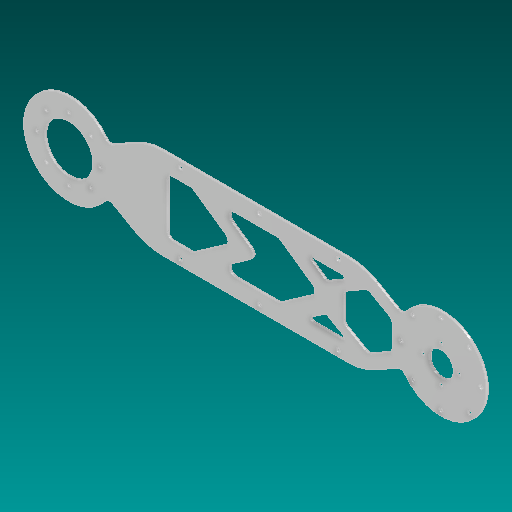
# Autodesk Inventor part: arm1 tweede kant
Saved by Autodesk Inventor 2020.3 (Build 243373000, 373)
## iProperties
Created: 2020-05-23
Part Number: arm1 tweede kant
Material: Aluminum 6061
Document SubType Name: Sheet Metal
Designer: Svend
Mass: 232.394 g
Surface Area: 513.63 cm^2
Volume: 86.0718 cm^3
Density: 2.7 g/cm^3
Sheet Metal Rule: Default_mm
Appearance: Aluminum - Polished
Author: Svend
Autodesk Inventor part; units mm, degrees
ref_plane "YZ Plane" through (0, 0, 0) normal (1, 0, 0) x (0, 1, 0)
ref_plane "XZ Plane" through (0, 0, 0) normal (0, 1, 0) x (-1, 0, 0)
ref_plane "XY Plane" through (0, 0, 0) normal (0, 0, 1) x (1, 0, 0)
sketch "Sketch1" plane through (0, 0, 0) normal (0, 0, 1) x (1, 0, 0)
  circle A0 centre (346.0004, 0) radius 1.55
  circle A1 centre (330, 0) radius 11
  arc A2 (51.9261, 10.7279) -> (51.9261, 14.7279) centre (51.9261, 12.7279) ccw
  line L0 (51.9261, 10.7279) -> (41.9261, 10.7279)
  arc A3 (41.9261, 14.7279) -> (41.9261, 10.7279) centre (41.9261, 12.7279) ccw
  line L1 (41.9261, 14.7279) -> (51.9261, 14.7279)
  arc A4 (77.3819, 10.7279) -> (77.3819, 14.7279) centre (77.3819, 12.7279) ccw
  line L2 (77.3819, 10.7279) -> (67.3819, 10.7279)
  arc A5 (67.3819, 14.7279) -> (67.3819, 10.7279) centre (67.3819, 12.7279) ccw
  line L3 (67.3819, 14.7279) -> (77.3819, 14.7279)
  arc A6 (51.9261, -14.7279) -> (51.9261, -10.7279) centre (51.9261, -12.7279) ccw
  line L4 (51.9261, -14.7279) -> (41.9261, -14.7279)
  arc A7 (41.9261, -10.7279) -> (41.9261, -14.7279) centre (41.9261, -12.7279) ccw
  line L5 (41.9261, -10.7279) -> (51.9261, -10.7279)
  arc A8 (67.3819, -10.7279) -> (67.3819, -14.7279) centre (67.3819, -12.7279) ccw
  line L6 (67.3819, -10.7279) -> (77.3819, -10.7279)
  arc A9 (77.3819, -14.7279) -> (77.3819, -10.7279) centre (77.3819, -12.7279) ccw
  line L7 (77.3819, -14.7279) -> (67.3819, -14.7279)
  circle A10 centre (59.654, 0) radius 8.5
  circle A11 centre (28, 0) radius 1.6
  line L8 (0, -40) -> (330, -40)
  arc A12 (330, -40) -> (330, 40) centre (330, 0) ccw
  line L9 (330, 40) -> (0, 40)
  arc A13 (0, 40) -> (0, -40) centre (0, 0) ccw
  line L10 (-4.8, -1) -> (-4.8, 1)
  line L11 (-4.8, 1) -> (-3.873, 1)
  arc A14 (-3.873, -1) -> (-3.873, 1) centre (0, 0) ccw
  line L12 (-3.873, -1) -> (-4.8, -1)
  circle A15 centre (0, 8) radius 2
  circle A16 centre (-6.9282, -4) radius 2
  circle A17 centre (6.9282, -4) radius 2
  circle A18 centre (19.799, 19.799) radius 1.6
  circle A19 centre (0, 28) radius 1.6
  circle A20 centre (-19.799, 19.799) radius 1.6
  circle A21 centre (-28, 0) radius 1.6
  circle A22 centre (-19.799, -19.799) radius 1.6
  circle A23 centre (0, -28) radius 1.6
  circle A24 centre (19.799, -19.799) radius 1.6
  circle A25 centre (330, 16.0004) radius 1.55
  circle A26 centre (313.9996, 0) radius 1.55
  circle A27 centre (330, -16.0004) radius 1.55
  line L13 (54.654, 0) -> (64.654, 0) construction
  line L14 (54.654, -8.5) -> (64.654, -8.5)
  line L15 (64.654, 8.5) -> (54.654, 8.5)
  arc A28 (54.654, 8.5) -> (54.654, -8.5) centre (54.654, 0) ccw
  arc A29 (64.654, -8.5) -> (64.654, 8.5) centre (64.654, 0) ccw
  circle A30 centre (0, 0) radius 21.5
  point P0 (-4.8, 0)
  point P1 (4, 0)
  point P2 (370, 0)
  dimension "d0" = 4
  dimension "d1" = 8.8
  dimension "d2" = 2
  dimension "d6" = 4
  dimension "d7" = 8
  dimension "d14" = 360
  dimension "d16" = 28
  dimension "d17" = 3.2
  dimension "d20" = 360
  dimension "d22" = 17
  dimension "d23" = 59.654
  dimension "d24" = 2
  dimension "d25" = 10
  dimension "d26" = 12.7279
  dimension "d27" = 17.7279
  dimension "d28" = 12.7279
  dimension "d29" = 17.7279
  dimension "d30" = 17.7279
  dimension "d31" = 17.7279
  dimension "d32" = 22
  dimension "d33" = 39.9999
  dimension "d35" = 3.1
  dimension "d36" = 16.0004
  dimension "d39" = 360
  dimension "d72" = 270.346
  dimension "d87" = 5
  dimension "d95" = 43
  measures "d0" radius of A14
  measures "d1" distance from line of point (4, 0) L10
  measures "d2" distance between parallel lines of L12 L11
  measures "d6" diameter of A15
  measures "d7" distance of A14.centre A15.centre
  measures "d16" distance of A14.centre A11.centre
  measures "d17" diameter of A11
  measures "d22" diameter of A10
  measures "d23" distance of A14.centre A10.centre
  measures "d24" radius of A3
  measures "d25" distance of L0.start L0.end
  measures "d26" vertical distance of A10.centre A2.centre
  measures "d27" horizontal distance of A10.centre A3.centre
  measures "d28" vertical distance of A8.centre A10.centre
  measures "d29" horizontal distance of A9.centre A10.centre
  measures "d30" horizontal distance of A7.centre A10.centre
  measures "d31" horizontal distance of A4.centre A10.centre
  measures "d32" diameter of A1
  measures "d33" radius of A13
  measures "d35" diameter of A0
  measures "d36" distance of A1.centre A0.centre
  measures "d72" distance of A1.centre A10.centre
  measures "d87" distance of A10.centre L13.end
  measures "d95" diameter of A30
extrude "Plate1" add sketch "Sketch1" along normal mid plane 2 contours L0 A3 L1 A2 | L2 A5 L3 A4 | L4 A7 L5 A6 | L6 A9 L7 A8 | A10 | A10 L15 A29 L14 | A10 L14 A28 L15 | A13 L9 A12 L8
sketch "Sketch2" plane through (0, 0, -1) normal (0, 0, -1) x (-1, 0, 0)
  circle A0 centre (-330, 0) radius 11 projected
  circle A1 centre (-19.799, -19.799) radius 1.6 projected
  circle A2 centre (0, -28) radius 1.6 projected
  circle A3 centre (19.799, -19.799) radius 1.6 projected
  circle A4 centre (28, 0) radius 1.6 projected
  circle A5 centre (19.799, 19.799) radius 1.6 projected
  circle A6 centre (0, 28) radius 1.6 projected
  circle A7 centre (-19.799, 19.799) radius 1.6 projected
  circle A8 centre (-28, 0) radius 1.6 projected
  circle A9 centre (-330, -16.0004) radius 1.55 projected
  circle A10 centre (-313.9996, 0) radius 1.55 projected
  circle A11 centre (-330, 16.0004) radius 1.55 projected
  circle A12 centre (-346.0004, 0) radius 1.55 projected
  line L0 (0, -40) -> (-330, -40) projected
  arc A13 (0, -40) -> (0, 40) centre (0, 0) ccw projected
  line L1 (-330, 40) -> (0, 40) projected
  arc A14 (-330, 40) -> (-330, -40) centre (-330, 0) ccw projected
  line L2 (-330, 40) -> (0, 40) projected
  arc A15 (-330, 40) -> (-330, -40) centre (-330, 0) ccw projected
  line L3 (-330, 0) -> (0, 0)
  line L4 (0, -40) -> (-330, -40) projected
  line L5 (-209.9233, -25) -> (-249.9233, -25)
  line L6 (-249.9233, -25) -> (-228, -12.3426)
  line L7 (-228, -12.3426) -> (-209.9233, -25)
  line L8 (-260.718, -40) -> (-295.359, -20)
  line L9 (-222, 0) -> (-186.2963, -25)
  line L10 (-186.2963, -25) -> (-131.2963, -25)
  line L11 (-131.2963, -25) -> (-167, 0)
  line L12 (-109.2963, -25) -> (-145, 0)
  line L13 (-87, -25) -> (-109.2963, -25)
  line L14 (-87, -25) -> (-87, 0)
  line L15 (-209.9233, 25) -> (-249.9233, 25)
  line L16 (-249.9233, 25) -> (-228, 12.3426)
  line L17 (-228, 12.3426) -> (-209.9233, 25)
  line L18 (-222, 0) -> (-186.2963, 25)
  line L19 (-186.2963, 25) -> (-131.2963, 25)
  line L20 (-131.2963, 25) -> (-167, 0)
  line L21 (-109.2963, 25) -> (-145, 0)
  line L22 (-87, 25) -> (-109.2963, 25)
  line L23 (-87, 25) -> (-87, 0)
  line L24 (-295.359, 20) -> (-260.718, 40)
  line L25 (-260.718, 40) -> (-330, 40)
  arc A16 (-295.359, 20) -> (-330, 40) centre (-330, 0) ccw
  arc A17 (-330, -40) -> (-295.359, -20) centre (-330, 0) ccw
  line L26 (-286.6506, -12.5) -> (-286.6506, 12.5)
  line L27 (-286.6506, 12.5) -> (-265, 25)
  line L28 (-265, 25) -> (-243.3494, 12.5)
  line L29 (-243.3494, 12.5) -> (-243.3494, -12.5)
  line L30 (-243.3494, -12.5) -> (-265, -25)
  line L31 (-265, -25) -> (-286.6506, -12.5)
  line L32 (-165, 40) -> (-165, -40)
  line L33 (0, 40) -> (-330, 40)
  line L34 (-69.282, -40) -> (-34.641, -20)
  arc A18 (-34.641, -20) -> (0, -40) centre (0, 0) ccw
  line L35 (-330, -40) -> (0, -40) projected
  line L36 (0, -40) -> (-69.282, -40)
  line L37 (-69.282, 40) -> (-34.641, 20)
  arc A19 (0, 40) -> (-34.641, 20) centre (0, 0) ccw
  line L38 (0, 40) -> (-69.282, 40)
  point P0 (-323.7858, 40)
  point P1 (-323.7858, -40)
  point P2 (-265, 0)
  point P3 (-228, 0)
  point P4 (-265, 0)
  dimension "d47" = 40
  dimension "d49" = 102
  dimension "d52" = 35
  dimension "d54" = 55
  dimension "d55" = 25
  dimension "d59" = 108
  dimension "d60" = 185
  dimension "d64" = 58
  dimension "d67" = 65
  constraints: 69 end point, 15 symmetric about line, 9 parallel, 9 point on line, 8 point on circle, 4 centre point, 4 collinear, 4 horizontal alignment, 4 line through centre, 3 coincident, 3 horizontal, 3 midpoint, 3 perpendicular, 3 tangent, 1 vertical alignment, 15 other
  measures "d47" distance of L5.start L5.end
  measures "d49" distance of A0.centre point (-228, 0)
  measures "d52" angle of L11 L10
  measures "d54" distance of L9.end L10.end
  measures "d55" distance between parallel lines of L3 L10
  measures "d59" distance of A0.centre L9.start
  measures "d60" distance of A0.centre L12.end
  measures "d64" distance from line of L14 L12.end
  measures "d67" distance of A0.centre point (-265, 0)
extrude "Cut1" cut sketch "Sketch2" against normal blind 2 contours L0 L34 A18 | A19 L37 L1 | L0 A17 L8 | L32 L11 L10 | L10 L9 L3 L11 L32 | L24 A16 L1 | L32 L20 L3 L18 L19 | L19 L20 L32 | L21 L22 L23 L3 | L3 L14 L13 L12 | L26 L27 L28 L29 L3 | L3 L29 L30 L31 L26 | L5 L6 L7 | L17 L16 L15
fillet "Fillet1" radius 2 6 edges at (249.9233, -25, 0) (209.9233, -25, 0) (228, -12.3426, 0) (249.9233, 25, 0) (228, 12.3426, 0) (209.9233, 25, 0)
fillet "Fillet2" radius 5 6 edges at (286.6506, -12.5, 0) (265, -25, 0) (243.3494, -12.5, 0) (243.3494, 12.5, 0) (265, 25, 0) (286.6506, 12.5, 0)
fillet "Fillet3" radius 5 11 edges at (222, 0, 0) (186.2963, -25, 0) (131.2963, -25, 0) (131.2963, 25, 0) (167, 0, 0) (186.2963, 25, 0) (145, 0, 0) (109.2963, -25, 0) (87, -25, 0) (87, 25, 0) (109.2963, 25, 0)
fillet "Fillet4" radius 50 4 edges at (260.718, -40, 0) (260.718, 40, 0) (69.282, 40, 0) (69.282, -40, 0)
fillet "Fillet5" radius 5 4 edges at (295.359, -20, 0) (295.359, 20, 0) (34.641, -20, 0) (34.641, 20, 0)
sketch "Sketch3" plane through (0, 0, -1) normal (0, 0, -1) x (-1, 0, 0)
  arc A0 (-82.6794, -40) -> (-57.6794, -33.3012) centre (-82.6794, 10) ccw projected
  line L0 (-57.6794, -33.3012) -> (-38.7298, -22.3607) projected
  arc A1 (-32.2043, -23.7251) -> (-38.7298, -22.3607) centre (-36.2298, -26.6908) ccw projected
  arc A2 (-32.2043, -23.7251) -> (-32.2043, 23.7251) centre (0, 0) ccw projected
  arc A3 (-38.7298, 22.3607) -> (-32.2043, 23.7251) centre (-36.2298, 26.6908) ccw projected
  line L1 (-38.7298, 22.3607) -> (-57.6794, 33.3012) projected
  arc A4 (-57.6794, 33.3012) -> (-82.6794, 40) centre (-82.6794, -10) ccw projected
  line L2 (-247.3206, 40) -> (-82.6794, 40) projected
  arc A5 (-247.3206, 40) -> (-272.3206, 33.3012) centre (-247.3206, -10) ccw projected
  line L3 (-272.3206, 33.3012) -> (-291.2702, 22.3607) projected
  arc A6 (-297.7957, 23.7251) -> (-291.2702, 22.3607) centre (-293.7702, 26.6908) ccw projected
  arc A7 (-297.7957, 23.7251) -> (-297.7957, -23.7251) centre (-330, 0) ccw projected
  arc A8 (-291.2702, -22.3607) -> (-297.7957, -23.7251) centre (-293.7702, -26.6908) ccw projected
  line L4 (-291.2702, -22.3607) -> (-272.3206, -33.3012) projected
  arc A9 (-272.3206, -33.3012) -> (-247.3206, -40) centre (-247.3206, 10) ccw projected
  line L5 (-82.6794, -40) -> (-247.3206, -40) projected
  arc A10 (-161.1506, 4.0958) -> (-161.1506, -4.0958) centre (-158.2828, 0) ccw projected
  line L6 (-161.1506, -4.0958) -> (-144.2864, -15.9042) projected
  arc A11 (-147.1543, -25) -> (-144.2864, -15.9042) centre (-147.1543, -20) ccw projected
  line L7 (-147.1543, -25) -> (-184.7198, -25) projected
  arc A12 (-187.5877, -24.0958) -> (-184.7198, -25) centre (-184.7198, -20) ccw projected
  line L8 (-187.5877, -24.0958) -> (-216.1506, -4.0958) projected
  arc A13 (-216.1506, 4.0958) -> (-216.1506, -4.0958) centre (-213.2828, 0) ccw projected
  line L9 (-216.1506, 4.0958) -> (-187.5877, 24.0958) projected
  arc A14 (-184.7198, 25) -> (-187.5877, 24.0958) centre (-184.7198, 20) ccw projected
  line L10 (-184.7198, 25) -> (-147.1543, 25) projected
  arc A15 (-144.2864, 15.9042) -> (-147.1543, 25) centre (-147.1543, 20) ccw projected
  line L11 (-144.2864, 15.9042) -> (-161.1506, 4.0958) projected
  line L12 (-215.1194, 21.3617) -> (-226.9563, 13.0734) projected
  arc A16 (-229.1034, 12.9796) -> (-226.9563, 13.0734) centre (-228.1034, 14.7117) ccw projected
  line L13 (-229.1034, 12.9796) -> (-243.4592, 21.2679) projected
  arc A17 (-242.4592, 25) -> (-243.4592, 21.2679) centre (-242.4592, 23) ccw projected
  line L14 (-242.4592, 25) -> (-216.2665, 25) projected
  arc A18 (-215.1194, 21.3617) -> (-216.2665, 25) centre (-216.2665, 23) ccw projected
  line L15 (-226.9563, -13.0734) -> (-215.1194, -21.3617) projected
  arc A19 (-216.2665, -25) -> (-215.1194, -21.3617) centre (-216.2665, -23) ccw projected
  line L16 (-216.2665, -25) -> (-242.4592, -25) projected
  arc A20 (-243.4592, -21.2679) -> (-242.4592, -25) centre (-242.4592, -23) ccw projected
  line L17 (-243.4592, -21.2679) -> (-229.1034, -12.9796) projected
  arc A21 (-226.9563, -13.0734) -> (-229.1034, -12.9796) centre (-228.1034, -14.7117) ccw projected
  line L18 (-267.5, -23.5566) -> (-284.1506, -13.9434) projected
  arc A22 (-286.6506, -9.6132) -> (-284.1506, -13.9434) centre (-281.6506, -9.6132) ccw projected
  line L19 (-286.6506, -9.6132) -> (-286.6506, 9.6132) projected
  arc A23 (-284.1506, 13.9434) -> (-286.6506, 9.6132) centre (-281.6506, 9.6132) ccw projected
  line L20 (-284.1506, 13.9434) -> (-267.5, 23.5566) projected
  arc A24 (-262.5, 23.5566) -> (-267.5, 23.5566) centre (-265, 19.2265) ccw projected
  line L21 (-262.5, 23.5566) -> (-245.8494, 13.9434) projected
  arc A25 (-243.3494, 9.6132) -> (-245.8494, 13.9434) centre (-248.3494, 9.6132) ccw projected
  line L22 (-243.3494, 9.6132) -> (-243.3494, -9.6132) projected
  arc A26 (-245.8494, -13.9434) -> (-243.3494, -9.6132) centre (-248.3494, -9.6132) ccw projected
  line L23 (-245.8494, -13.9434) -> (-262.5, -23.5566) projected
  arc A27 (-267.5, -23.5566) -> (-262.5, -23.5566) centre (-265, -19.2265) ccw projected
  line L24 (-92, -25) -> (-107.7198, -25) projected
  arc A28 (-110.5877, -24.0958) -> (-107.7198, -25) centre (-107.7198, -20) ccw projected
  line L25 (-110.5877, -24.0958) -> (-139.1506, -4.0958) projected
  arc A29 (-139.1506, 4.0958) -> (-139.1506, -4.0958) centre (-136.2828, 0) ccw projected
  line L26 (-139.1506, 4.0958) -> (-110.5877, 24.0958) projected
  arc A30 (-107.7198, 25) -> (-110.5877, 24.0958) centre (-107.7198, 20) ccw projected
  line L27 (-107.7198, 25) -> (-92, 25) projected
  arc A31 (-87, 20) -> (-92, 25) centre (-92, 20) ccw projected
  line L28 (-87, 20) -> (-87, -20) projected
  arc A32 (-92, -25) -> (-87, -20) centre (-92, -20) ccw projected
  circle A33 centre (-330, 0) radius 11 projected
  circle A34 centre (-19.799, -19.799) radius 1.6 projected
  circle A35 centre (0, -28) radius 1.6 projected
  circle A36 centre (19.799, -19.799) radius 1.6 projected
  circle A37 centre (28, 0) radius 1.6 projected
  circle A38 centre (19.799, 19.799) radius 1.6 projected
  circle A39 centre (0, 28) radius 1.6 projected
  circle A40 centre (-19.799, 19.799) radius 1.6 projected
  circle A41 centre (-28, 0) radius 1.6 projected
  circle A42 centre (-330, -16.0004) radius 1.55 projected
  circle A43 centre (-313.9996, 0) radius 1.55 projected
  circle A44 centre (-330, 16.0004) radius 1.55 projected
  circle A45 centre (-346.0004, 0) radius 1.55 projected
  circle A46 centre (-365.5, 0) radius 1.6
  circle A47 centre (-355.1023, -25.1023) radius 1.6
  circle A48 centre (-330, -35.5) radius 1.6
  circle A49 centre (-304.8977, -25.1023) radius 1.6
  circle A50 centre (-294.5, 0) radius 1.6
  circle A51 centre (-304.8977, 25.1023) radius 1.6
  circle A52 centre (-330, 35.5) radius 1.6
  circle A53 centre (-355.1023, 25.1023) radius 1.6
  point P0 (0, 0)
  dimension "d73" = 3.2
  dimension "d74" = 35.5
  dimension "d77" = 360
  constraints: 8 centre point, 1 horizontal alignment, 17 other
  measures "d73" diameter of A46
  measures "d74" distance of A33.centre A46.centre
chamfer "Chamfer2" distance 1.5 angle 45 4 edges at (344.4504, 0, -1) (328.45, 16.0004, -1) (312.4496, 0, -1) (328.45, -16.0004, -1)
hole "Hole1" at (330, -35.5, -1) at (355.1023, -25.1023, -1) at (365.5, 0, -1) at (355.1023, 25.1023, -1) at (330, 35.5, -1) at (304.8977, 25.1023, -1) at (294.5, 0, -1) at (304.8977, -25.1023, -1) direction (0, 0, 1) diameter 4 end through all clearance for "Countersunk Flat Head Screw ISO 2009/7046" size "M4" standard "ISO"
sketch "Sketch4" plane through (0, 0, -1) normal (0, 0, -1) x (-1, 0, 0)
  circle A0 centre (-169, 35) radius 2.1 projected
  circle A1 centre (-239, -35) radius 2.1 projected
  circle A2 centre (-99, -35) radius 2.1 projected
  circle A3 centre (-169, -35) radius 2.1 projected
  circle A4 centre (-99, 35) radius 2.1 projected
  circle A5 centre (-239, 35) radius 2.1 projected
  circle A6 centre (-294.5, 0) radius 2 projected
  circle A7 centre (-330, -35.5) radius 2 projected
  circle A8 centre (-365.5, 0) radius 2 projected
  circle A9 centre (-330, 35.5) radius 2 projected
  circle A10 centre (-355.1023, 25.1023) radius 2 projected
  circle A11 centre (-355.1023, -25.1023) radius 2 projected
  circle A12 centre (-304.8977, -25.1023) radius 2 projected
  circle A13 centre (-304.8977, 25.1023) radius 2 projected
  arc A14 (-57.6794, 33.3012) -> (-82.6794, 40) centre (-82.6794, -10) ccw projected
  line L0 (-247.3206, 40) -> (-82.6794, 40) projected
  arc A15 (-247.3206, 40) -> (-272.3206, 33.3012) centre (-247.3206, -10) ccw projected
  line L1 (-272.3206, 33.3012) -> (-291.2702, 22.3607) projected
  arc A16 (-297.7957, 23.7251) -> (-291.2702, 22.3607) centre (-293.7702, 26.6908) ccw projected
  arc A17 (-297.7957, 23.7251) -> (-297.7957, -23.7251) centre (-330, 0) ccw projected
  arc A18 (-291.2702, -22.3607) -> (-297.7957, -23.7251) centre (-293.7702, -26.6908) ccw projected
  line L2 (-291.2702, -22.3607) -> (-272.3206, -33.3012) projected
  arc A19 (-272.3206, -33.3012) -> (-247.3206, -40) centre (-247.3206, 10) ccw projected
  line L3 (-82.6794, -40) -> (-247.3206, -40) projected
  arc A20 (-82.6794, -40) -> (-57.6794, -33.3012) centre (-82.6794, 10) ccw projected
  line L4 (-57.6794, -33.3012) -> (-38.7298, -22.3607) projected
  arc A21 (-32.2043, -23.7251) -> (-38.7298, -22.3607) centre (-36.2298, -26.6908) ccw projected
  arc A22 (-32.2043, -23.7251) -> (-32.2043, 23.7251) centre (0, 0) ccw projected
  arc A23 (-38.7298, 22.3607) -> (-32.2043, 23.7251) centre (-36.2298, 26.6908) ccw projected
  line L5 (-38.7298, 22.3607) -> (-57.6794, 33.3012) projected
  line L6 (-226.9563, -13.0734) -> (-215.1194, -21.3617) projected
  arc A24 (-216.2665, -25) -> (-215.1194, -21.3617) centre (-216.2665, -23) ccw projected
  line L7 (-216.2665, -25) -> (-242.4592, -25) projected
  arc A25 (-243.4592, -21.2679) -> (-242.4592, -25) centre (-242.4592, -23) ccw projected
  line L8 (-243.4592, -21.2679) -> (-229.1034, -12.9796) projected
  arc A26 (-226.9563, -13.0734) -> (-229.1034, -12.9796) centre (-228.1034, -14.7117) ccw projected
  arc A27 (-161.1506, 4.0958) -> (-161.1506, -4.0958) centre (-158.2828, 0) ccw projected
  line L9 (-161.1506, -4.0958) -> (-144.2864, -15.9042) projected
  arc A28 (-147.1543, -25) -> (-144.2864, -15.9042) centre (-147.1543, -20) ccw projected
  line L10 (-147.1543, -25) -> (-184.7198, -25) projected
  arc A29 (-187.5877, -24.0958) -> (-184.7198, -25) centre (-184.7198, -20) ccw projected
  line L11 (-187.5877, -24.0958) -> (-216.1506, -4.0958) projected
  arc A30 (-216.1506, 4.0958) -> (-216.1506, -4.0958) centre (-213.2828, 0) ccw projected
  line L12 (-216.1506, 4.0958) -> (-187.5877, 24.0958) projected
  arc A31 (-184.7198, 25) -> (-187.5877, 24.0958) centre (-184.7198, 20) ccw projected
  line L13 (-184.7198, 25) -> (-147.1543, 25) projected
  arc A32 (-144.2864, 15.9042) -> (-147.1543, 25) centre (-147.1543, 20) ccw projected
  line L14 (-144.2864, 15.9042) -> (-161.1506, 4.0958) projected
  line L15 (-215.1194, 21.3617) -> (-226.9563, 13.0734) projected
  arc A33 (-229.1034, 12.9796) -> (-226.9563, 13.0734) centre (-228.1034, 14.7117) ccw projected
  line L16 (-229.1034, 12.9796) -> (-243.4592, 21.2679) projected
  arc A34 (-242.4592, 25) -> (-243.4592, 21.2679) centre (-242.4592, 23) ccw projected
  line L17 (-242.4592, 25) -> (-216.2665, 25) projected
  arc A35 (-215.1194, 21.3617) -> (-216.2665, 25) centre (-216.2665, 23) ccw projected
  line L18 (-284.1506, 13.9434) -> (-267.5, 23.5566) projected
  arc A36 (-262.5, 23.5566) -> (-267.5, 23.5566) centre (-265, 19.2265) ccw projected
  line L19 (-262.5, 23.5566) -> (-245.8494, 13.9434) projected
  arc A37 (-243.3494, 9.6132) -> (-245.8494, 13.9434) centre (-248.3494, 9.6132) ccw projected
  line L20 (-243.3494, 9.6132) -> (-243.3494, -9.6132) projected
  arc A38 (-245.8494, -13.9434) -> (-243.3494, -9.6132) centre (-248.3494, -9.6132) ccw projected
  line L21 (-245.8494, -13.9434) -> (-262.5, -23.5566) projected
  arc A39 (-267.5, -23.5566) -> (-262.5, -23.5566) centre (-265, -19.2265) ccw projected
  line L22 (-267.5, -23.5566) -> (-284.1506, -13.9434) projected
  arc A40 (-286.6506, -9.6132) -> (-284.1506, -13.9434) centre (-281.6506, -9.6132) ccw projected
  line L23 (-286.6506, -9.6132) -> (-286.6506, 9.6132) projected
  arc A41 (-284.1506, 13.9434) -> (-286.6506, 9.6132) centre (-281.6506, 9.6132) ccw projected
  line L24 (-107.7198, 25) -> (-92, 25) projected
  arc A42 (-87, 20) -> (-92, 25) centre (-92, 20) ccw projected
  line L25 (-87, 20) -> (-87, -20) projected
  arc A43 (-92, -25) -> (-87, -20) centre (-92, -20) ccw projected
  line L26 (-92, -25) -> (-107.7198, -25) projected
  arc A44 (-110.5877, -24.0958) -> (-107.7198, -25) centre (-107.7198, -20) ccw projected
  line L27 (-110.5877, -24.0958) -> (-139.1506, -4.0958) projected
  arc A45 (-139.1506, 4.0958) -> (-139.1506, -4.0958) centre (-136.2828, 0) ccw projected
  line L28 (-139.1506, 4.0958) -> (-110.5877, 24.0958) projected
  arc A46 (-107.7198, 25) -> (-110.5877, 24.0958) centre (-107.7198, 20) ccw projected
  arc A47 (-54.654, -8.5) -> (-54.654, 8.5) centre (-54.654, 0) ccw projected
  line L29 (-54.654, -8.5) -> (-64.654, -8.5) projected
  arc A48 (-64.654, 8.5) -> (-64.654, -8.5) centre (-64.654, 0) ccw projected
  line L30 (-64.654, 8.5) -> (-54.654, 8.5) projected
  circle A49 centre (-330, 0) radius 11 projected
  line L31 (-67.3819, 10.7279) -> (-77.3819, 10.7279) projected
  arc A50 (-77.3819, 14.7279) -> (-77.3819, 10.7279) centre (-77.3819, 12.7279) ccw projected
  line L32 (-77.3819, 14.7279) -> (-67.3819, 14.7279) projected
  arc A51 (-67.3819, 10.7279) -> (-67.3819, 14.7279) centre (-67.3819, 12.7279) ccw projected
  line L33 (-51.9261, 14.7279) -> (-41.9261, 14.7279) projected
  arc A52 (-41.9261, 10.7279) -> (-41.9261, 14.7279) centre (-41.9261, 12.7279) ccw projected
  line L34 (-41.9261, 10.7279) -> (-51.9261, 10.7279) projected
  arc A53 (-51.9261, 14.7279) -> (-51.9261, 10.7279) centre (-51.9261, 12.7279) ccw projected
  line L35 (-77.3819, -10.7279) -> (-67.3819, -10.7279) projected
  arc A54 (-67.3819, -14.7279) -> (-67.3819, -10.7279) centre (-67.3819, -12.7279) ccw projected
  line L36 (-67.3819, -14.7279) -> (-77.3819, -14.7279) projected
  arc A55 (-77.3819, -10.7279) -> (-77.3819, -14.7279) centre (-77.3819, -12.7279) ccw projected
  line L37 (-51.9261, -10.7279) -> (-41.9261, -10.7279) projected
  arc A56 (-41.9261, -14.7279) -> (-41.9261, -10.7279) centre (-41.9261, -12.7279) ccw projected
  line L38 (-41.9261, -14.7279) -> (-51.9261, -14.7279) projected
  arc A57 (-51.9261, -10.7279) -> (-51.9261, -14.7279) centre (-51.9261, -12.7279) ccw projected
  line L39 (4.8, -1) -> (3.873, -1) projected
  arc A58 (3.873, 1) -> (3.873, -1) centre (0, 0) ccw projected
  line L40 (3.873, 1) -> (4.8, 1) projected
  line L41 (4.8, 1) -> (4.8, -1) projected
  circle A59 centre (-6.9282, 4) radius 2 projected
  circle A60 centre (6.9282, 4) radius 2 projected
  circle A61 centre (0, -8) radius 2 projected
  circle A62 centre (-19.799, 19.799) radius 1.6 projected
  circle A63 centre (0, 28) radius 1.6 projected
  circle A64 centre (19.799, 19.799) radius 1.6 projected
  circle A65 centre (28, 0) radius 1.6 projected
  circle A66 centre (19.799, -19.799) radius 1.6 projected
  circle A67 centre (0, -28) radius 1.6 projected
  circle A68 centre (-19.799, -19.799) radius 1.6 projected
  circle A69 centre (-28, 0) radius 1.6 projected
  circle A70 centre (-330, 16.0004) radius 1.55 projected
  circle A71 centre (-313.9996, 0) radius 1.55 projected
  circle A72 centre (-330, -16.0004) radius 1.55 projected
  circle A73 centre (-346.0004, 0) radius 1.55 projected
  point P0 (0, 0)
  point P1 (-99, -35)
  point P2 (-169, -35)
  point P3 (-239, -35)
  point P4 (-239, 35)
  point P5 (-169, 35)
  point P6 (-99, 35)
  constraints: 6 coincident
hole "Hole2" at (99, -35, -1) at (169, -35, -1) at (239, -35, -1) at (239, 35, -1) at (169, 35, -1) at (99, 35, -1) direction (0, 0, 1) diameter 4.2 end through all clearance for "Countersunk Flat Head Screw ISO 2009/7046" size "M4" standard "ISO"
equation "\"d41\" = Thickness"
equation "\"BendRadius\" = Thickness"
equation "\"BendReliefWidth\" = Thickness"
equation "\"CornerReliefSize\" = 4 * Thickness"
equation "\"TransitionRadius\" = BendRadius"
equation "\"JacobiRadiusSize\" = BendRadius"
equation "\"GapSize\" = Thickness"
equation "\"Thickness\" = 2"
body "Solid1"
